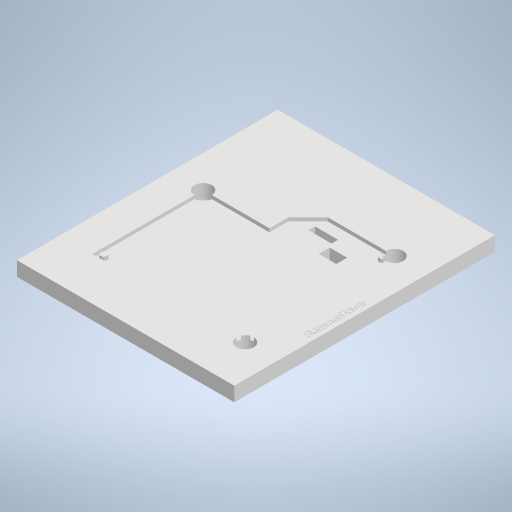
# Autodesk Inventor part: _Tooling_PCBPaste
Saved by Autodesk Inventor 2023.2 (Build 272271000, 271)
## iProperties
Created: 2023-03-08
Part Number: _Tooling_PCBPaste
Material: Generic
Document SubType Name: Modeling
Designer: atrus
Density: 1 g/cm^3
Appearance: Default
Author: atrus
Autodesk Inventor part; units mm, degrees
ref_plane "YZ Plane" through (0, 0, 0) normal (1, 0, 0) x (0, 1, 0)
ref_plane "XZ Plane" through (0, 0, 0) normal (0, 1, 0) x (-1, 0, 0)
ref_plane "XY Plane" through (0, 0, 0) normal (0, 0, 1) x (1, 0, 0)
sketch "Sketch1" plane through (0, 0, 0) normal (0, 1, 0) x (-1, 0, 0)
  line L0 (0, 0) -> (-100, 0)
  line L1 (-100, 0) -> (-100, -120)
  line L2 (-100, -120) -> (0, -120)
  line L3 (0, -120) -> (0, 0)
  dimension "d0" = 120
  dimension "d1" = 100
  constraints: 8 end point, 2 parallel, 1 horizontal, 1 perpendicular
  measures "d0" distance of L2.end L0.start
  measures "d1" distance of L0.start L0.end
extrude "Extrusion1" add sketch "Sketch1" along normal blind 5
sketch "Sketch2" plane through (0, 5, 0) normal (0, 1, 0) x (1, 0, 0)
  circle A0 centre (71.8797, 76.0683) radius 0.45 construction
  circle A1 centre (66.7997, 75.0523) radius 0.45 construction
  circle A2 centre (66.7997, 77.0843) radius 0.45 construction
  circle A3 centre (54.9887, 82.1643) radius 0.508 construction
  circle A4 centre (57.5287, 82.1643) radius 0.508 construction
  circle A5 centre (60.0687, 82.1643) radius 0.508 construction
  circle A6 centre (62.6087, 82.1643) radius 0.508 construction
  circle A7 centre (82.5477, 85.7203) radius 1.6256 construction
  circle A8 centre (82.5477, 22.7283) radius 1.6256 construction
  circle A9 centre (17.5237, 22.4743) radius 1.6256 construction
  circle A10 centre (78.7377, 80.8943) radius 0.425 construction
  circle A11 centre (66.0377, 83.4343) radius 0.425 construction
  line L0 (14.9837, 70.7343) -> (14.9837, 19.9343) construction
  line L1 (14.9837, 19.9343) -> (85.0877, 19.9343) construction
  line L2 (85.0877, 19.9343) -> (85.0877, 88.5143) construction
  line L3 (85.0877, 88.5143) -> (54.3537, 88.5143) construction
  line L4 (54.3537, 88.5143) -> (45.4637, 79.6243) construction
  line L5 (45.4637, 79.6243) -> (45.4637, 70.7343) construction
  line L6 (45.4637, 70.7343) -> (14.9837, 70.7343) construction
  line L7 (14.8837, 70.8343) -> (14.8837, 19.8343)
  line L8 (14.8837, 19.8343) -> (85.1877, 19.8343)
  line L9 (85.1877, 19.8343) -> (85.1877, 88.6143)
  line L10 (85.1877, 88.6143) -> (54.3123, 88.6143)
  line L11 (54.3123, 88.6143) -> (45.3637, 79.6658)
  line L12 (45.3637, 79.6658) -> (45.3637, 70.8343)
  line L13 (45.3637, 70.8343) -> (14.8837, 70.8343)
  circle A12 centre (82.5477, 85.7203) radius 1.5256
  circle A13 centre (17.5237, 22.4743) radius 1.5256
  circle A14 centre (82.5477, 22.7283) radius 1.5256
  line L14 (100, 120) -> (0, 120) projected
  line L15 (100, 0) -> (100, 120) projected
  line L16 (0, 120) -> (100, 120)
  line L17 (100, 120) -> (100, 0)
  line L18 (100, 0) -> (0, 0)
  line L19 (0, 0) -> (0, 120)
  point P0 (0, 0)
  dimension "d4" = 0.1
  dimension "d5" = 0.1
  dimension "d6" = 0.1
  dimension "d7" = 0.1
  constraints: 22 end point, 3 centre point, 2 parallel, 1 horizontal, 1 perpendicular, 6 other
  measures "d4" distance between parallel lines of L6 L13
  measures "d5" radial gap between concentric circles of A7 A12
  measures "d6" radial gap between concentric circles of A9 A13
  measures "d7" radial gap between concentric circles of A8 A14
extrude "Extrusion2" add sketch "Sketch2" along normal blind 1.6
sketch "Sketch3" plane through (0, 6.6, 0) normal (0, 1, 0) x (1, 0, 0)
  line L0 (45.3637, 70.8343) -> (14.8837, 70.8343) projected
  circle A0 centre (14.8837, 70.8343) radius 4
  line L1 (85.1877, 88.6143) -> (54.3123, 88.6143) projected
  circle A1 centre (85.1877, 88.6143) radius 4
  line L2 (85.1877, 19.8343) -> (14.8837, 19.8343) projected
  circle A2 centre (85.1877, 19.8343) radius 4
  circle A3 centre (54.9887, 82.1643) radius 0.508 construction
  circle A4 centre (62.6087, 82.1643) radius 0.508 construction
  circle A5 centre (66.7997, 77.0843) radius 0.45 construction
  circle A6 centre (71.8797, 76.0683) radius 0.45 construction
  circle A7 centre (66.7997, 75.0523) radius 0.45 construction
  line L3 (53.4887, 83.6643) -> (64.1087, 83.6643)
  line L4 (64.1087, 83.6643) -> (64.1087, 80.6643)
  line L5 (64.1087, 80.6643) -> (53.4887, 80.6643)
  line L6 (53.4887, 80.6643) -> (53.4887, 83.6643)
  line L7 (65.2997, 78.5843) -> (73.3797, 78.5843)
  line L8 (73.3797, 78.5843) -> (73.3797, 73.5523)
  line L9 (73.3797, 73.5523) -> (65.2997, 73.5523)
  line L10 (65.2997, 73.5523) -> (65.2997, 78.5843)
  point P0 (0, 0)
  point P1 (53.4887, 82.1643)
  point P2 (64.1087, 82.1643)
  point P3 (73.3797, 76.0683)
  dimension "d10" = 8
  dimension "d11" = 1.5
  dimension "d12" = 1.5
  dimension "d13" = 1.5
  dimension "d14" = 1.5
  dimension "d15" = 1.5
  dimension "d16" = 1.5
  dimension "d17" = 1.5
  dimension "d18" = 1.5
  constraints: 16 end point, 4 parallel, 3 centre point, 3 midpoint, 2 equal radius, 2 horizontal, 2 perpendicular
  measures "d10" diameter of A0
  measures "d11" distance of point (53.489, 82.164) A3.centre
  measures "d12" distance of point (64.109, 82.164) A4.centre
  measures "d13" distance from line of L5 A4.centre
  measures "d14" distance from line of L3 A3.centre
  measures "d15" distance from line of L7 A5.centre
  measures "d16" distance from line of L9 A7.centre
  measures "d17" distance from line of L10 A7.centre
  measures "d18" distance of point (73.38, 76.068) A6.centre
extrude "Extrusion3" cut sketch "Sketch3" against normal through all
sketch "Sketch4" plane through (0, 6.6, 0) normal (0, 1, 0) x (1, 0, 0)
  line L0 (94.8886, 36.1606) -> (94.8886, 63.4147) construction
  line L1 (94.8886, 63.4147) -> (98.1268, 63.4147) construction
  line L2 (98.1268, 63.4147) -> (98.1268, 36.1606) construction
  line L3 (98.1268, 36.1606) -> (94.8886, 36.1606) construction
  spline S0 degree 2 poles (98.1268, 37.319) (98.1268, 36.988) (97.9885, 36.5237) (97.8897, 36.3186) knots 0 0 0 1 2 2 2
  line L4 (97.8897, 36.3186) -> (97.3809, 36.3186)
  line L5 (97.3809, 36.3186) -> (97.3809, 36.3483)
  spline S1 degree 2 poles (97.3809, 36.3483) (97.5686, 36.5484) (97.7761, 37.0547) (97.7761, 37.2894) knots 0 0 0 1 2 2 2
  spline S2 degree 2 poles (97.7761, 37.2894) (97.7761, 37.6253) (97.4969, 37.9686) (97.2672, 37.9686) knots 0 0 0 1 2 2 2
  spline S3 degree 2 poles (97.2672, 37.9686) (97.0845, 37.9686) (96.8572, 37.7883) (96.8004, 37.5932) knots 0 0 0 1 2 2 2
  spline S4 degree 2 poles (96.8004, 37.5932) (96.7609, 37.4524) (96.7065, 37.2177) (96.6621, 37.0424) knots 0 0 0 1 2 2 2
  spline S5 degree 2 poles (96.6621, 37.0424) (96.6201, 36.8843) (96.4941, 36.6348) (96.3928, 36.5385) knots 0 0 0 1 2 2 2
  spline S6 degree 2 poles (96.3928, 36.5385) (96.2916, 36.4446) (96.0199, 36.3409) (95.842, 36.3409) knots 0 0 0 1 2 2 2
  spline S7 degree 2 poles (95.842, 36.3409) (95.4715, 36.3409) (94.9701, 36.9189) (94.9701, 37.3659) knots 0 0 0 1 2 2 2
  spline S8 degree 2 poles (94.9701, 37.3659) (94.9701, 37.6228) (95.0714, 38.0773) (95.1677, 38.2724) knots 0 0 0 1 2 2 2
  line L6 (95.1677, 38.2724) -> (95.6518, 38.2724)
  line L7 (95.6518, 38.2724) -> (95.6518, 38.2428)
  spline S9 degree 2 poles (95.6518, 38.2428) (95.5185, 38.0971) (95.3209, 37.6426) (95.3209, 37.3931) knots 0 0 0 1 2 2 2
  spline S10 degree 2 poles (95.3209, 37.3931) (95.3209, 37.1115) (95.5852, 36.7632) (95.8, 36.7632) knots 0 0 0 1 2 2 2
  spline S11 degree 2 poles (95.8, 36.7632) (95.9927, 36.7632) (96.2224, 36.9683) (96.2743, 37.1609) knots 0 0 0 1 2 2 2
  spline S12 degree 2 poles (96.2743, 37.1609) (96.3089, 37.2894) (96.3978, 37.6623) (96.4348, 37.7858) knots 0 0 0 1 2 2 2
  spline S13 degree 2 poles (96.4348, 37.7858) (96.5312, 38.0995) (96.919, 38.391) (97.203, 38.391) knots 0 0 0 1 2 2 2
  spline S14 degree 2 poles (97.203, 38.391) (97.3833, 38.391) (97.7291, 38.2453) (97.8502, 38.1143) knots 0 0 0 1 2 2 2
  spline S15 degree 2 poles (97.8502, 38.1143) (97.9835, 37.9686) (98.1268, 37.5981) (98.1268, 37.319) knots 0 0 0 1 2 2 2
  line L8 (98.0725, 40.6683) -> (98.0725, 40.162)
  line L9 (98.0725, 40.162) -> (96.9684, 39.3123)
  line L10 (96.9684, 39.3123) -> (97.1166, 39.1592)
  line L11 (97.1166, 39.1592) -> (98.0725, 39.1592)
  line L12 (98.0725, 39.1592) -> (98.0725, 38.7738)
  line L13 (98.0725, 38.7738) -> (94.8886, 38.7738)
  line L14 (94.8886, 38.7738) -> (94.8886, 39.1592)
  line L15 (94.8886, 39.1592) -> (96.751, 39.1592)
  line L16 (96.751, 39.1592) -> (95.7852, 40.0632)
  line L17 (95.7852, 40.0632) -> (95.7852, 40.5424)
  line L18 (95.7852, 40.5424) -> (96.7411, 39.6038)
  line L19 (96.7411, 39.6038) -> (98.0725, 40.6683)
  line L20 (98.0725, 41.2537) -> (98.0725, 40.8684)
  line L21 (98.0725, 40.8684) -> (95.7852, 40.8684)
  line L22 (95.7852, 40.8684) -> (95.7852, 41.2537)
  line L23 (95.7852, 41.2537) -> (98.0725, 41.2537)
  line L24 (95.4048, 41.2809) -> (95.4048, 40.8437)
  line L25 (95.4048, 40.8437) -> (95.0047, 40.8437)
  line L26 (95.0047, 40.8437) -> (95.0047, 41.2809)
  line L27 (95.0047, 41.2809) -> (95.4048, 41.2809)
  line L28 (98.0725, 44.4129) -> (96.7485, 44.4129)
  spline S16 degree 2 poles (96.7485, 44.4129) (96.5904, 44.4129) (96.3212, 44.3882) (96.2471, 44.3487) knots 0 0 0 1 2 2 2
  spline S17 degree 2 poles (96.2471, 44.3487) (96.1656, 44.3091) (96.0866, 44.1585) (96.0866, 44.0276) knots 0 0 0 1 2 2 2
  spline S18 degree 2 poles (96.0866, 44.0276) (96.0866, 43.909) (96.2323, 43.6373) (96.3706, 43.494) knots 0 0 0 1 2 2 2
  spline S19 degree 2 poles (96.3706, 43.494) (96.4052, 43.4965) (96.5015, 43.5014) (96.5657, 43.5014) knots 0 0 0 1 2 2 2
  line L29 (96.5657, 43.5014) -> (98.0725, 43.5014)
  line L30 (98.0725, 43.5014) -> (98.0725, 43.1161)
  line L31 (98.0725, 43.1161) -> (96.7485, 43.1161)
  spline S20 degree 2 poles (96.7485, 43.1161) (96.5904, 43.1161) (96.3212, 43.0914) (96.2471, 43.0519) knots 0 0 0 1 2 2 2
  spline S21 degree 2 poles (96.2471, 43.0519) (96.1656, 43.0124) (96.0866, 42.8617) (96.0866, 42.7308) knots 0 0 0 1 2 2 2
  spline S22 degree 2 poles (96.0866, 42.7308) (96.0866, 42.6073) (96.2422, 42.3331) (96.3632, 42.2047) knots 0 0 0 1 2 2 2
  line L32 (96.3632, 42.2047) -> (98.0725, 42.2047)
  line L33 (98.0725, 42.2047) -> (98.0725, 41.8194)
  line L34 (98.0725, 41.8194) -> (95.7852, 41.8194)
  line L35 (95.7852, 41.8194) -> (95.7852, 42.2047)
  line L36 (95.7852, 42.2047) -> (96.0372, 42.2047)
  spline S23 degree 2 poles (96.0372, 42.2047) (95.8865, 42.3554) (95.721, 42.6518) (95.721, 42.8296) knots 0 0 0 1 2 2 2
  spline S24 degree 2 poles (95.721, 42.8296) (95.721, 43.0321) (95.9063, 43.3458) (96.1162, 43.4273) knots 0 0 0 1 2 2 2
  spline S25 degree 2 poles (96.1162, 43.4273) (95.9211, 43.6027) (95.721, 43.9337) (95.721, 44.1264) knots 0 0 0 1 2 2 2
  spline S26 degree 2 poles (95.721, 44.1264) (95.721, 44.2746) (95.8124, 44.5166) (95.9161, 44.6055) knots 0 0 0 1 2 2 2
  spline S27 degree 2 poles (95.9161, 44.6055) (96.0199, 44.6969) (96.3311, 44.7982) (96.5657, 44.7982) knots 0 0 0 1 2 2 2
  line L37 (96.5657, 44.7982) -> (98.0725, 44.7982)
  line L38 (98.0725, 44.7982) -> (98.0725, 44.4129)
  line L39 (98.0725, 47.9327) -> (96.7485, 47.9327)
  spline S28 degree 2 poles (96.7485, 47.9327) (96.5904, 47.9327) (96.3212, 47.908) (96.2471, 47.8684) knots 0 0 0 1 2 2 2
  spline S29 degree 2 poles (96.2471, 47.8684) (96.1656, 47.8289) (96.0866, 47.6782) (96.0866, 47.5473) knots 0 0 0 1 2 2 2
  spline S30 degree 2 poles (96.0866, 47.5473) (96.0866, 47.4288) (96.2323, 47.1571) (96.3706, 47.0138) knots 0 0 0 1 2 2 2
  spline S31 degree 2 poles (96.3706, 47.0138) (96.4052, 47.0163) (96.5015, 47.0212) (96.5657, 47.0212) knots 0 0 0 1 2 2 2
  line L40 (96.5657, 47.0212) -> (98.0725, 47.0212)
  line L41 (98.0725, 47.0212) -> (98.0725, 46.6359)
  line L42 (98.0725, 46.6359) -> (96.7485, 46.6359)
  spline S32 degree 2 poles (96.7485, 46.6359) (96.5904, 46.6359) (96.3212, 46.6112) (96.2471, 46.5717) knots 0 0 0 1 2 2 2
  spline S33 degree 2 poles (96.2471, 46.5717) (96.1656, 46.5322) (96.0866, 46.3815) (96.0866, 46.2506) knots 0 0 0 1 2 2 2
  spline S34 degree 2 poles (96.0866, 46.2506) (96.0866, 46.1271) (96.2422, 45.8529) (96.3632, 45.7245) knots 0 0 0 1 2 2 2
  line L43 (96.3632, 45.7245) -> (98.0725, 45.7245)
  line L44 (98.0725, 45.7245) -> (98.0725, 45.3391)
  line L45 (98.0725, 45.3391) -> (95.7852, 45.3391)
  line L46 (95.7852, 45.3391) -> (95.7852, 45.7245)
  line L47 (95.7852, 45.7245) -> (96.0372, 45.7245)
  spline S35 degree 2 poles (96.0372, 45.7245) (95.8865, 45.8751) (95.721, 46.1715) (95.721, 46.3494) knots 0 0 0 1 2 2 2
  spline S36 degree 2 poles (95.721, 46.3494) (95.721, 46.5519) (95.9063, 46.8656) (96.1162, 46.9471) knots 0 0 0 1 2 2 2
  spline S37 degree 2 poles (96.1162, 46.9471) (95.9211, 47.1225) (95.721, 47.4535) (95.721, 47.6461) knots 0 0 0 1 2 2 2
  spline S38 degree 2 poles (95.721, 47.6461) (95.721, 47.7943) (95.8124, 48.0364) (95.9161, 48.1253) knots 0 0 0 1 2 2 2
  spline S39 degree 2 poles (95.9161, 48.1253) (96.0199, 48.2167) (96.3311, 48.318) (96.5657, 48.318) knots 0 0 0 1 2 2 2
  line L48 (96.5657, 48.318) -> (98.0725, 48.318)
  line L49 (98.0725, 48.318) -> (98.0725, 47.9327)
  spline S40 degree 2 poles (98.1243, 49.8519) (98.1243, 49.3035) (97.5093, 48.7008) (96.9412, 48.7008) knots 0 0 0 1 2 2 2
  spline S41 degree 2 poles (96.9412, 48.7008) (96.383, 48.7008) (95.721, 49.2862) (95.721, 49.758) knots 0 0 0 1 2 2 2
  spline S42 degree 2 poles (95.721, 49.758) (95.721, 49.9704) (95.8445, 50.2989) (95.9754, 50.42) knots 0 0 0 1 2 2 2
  spline S43 degree 2 poles (95.9754, 50.42) (96.1063, 50.5435) (96.4842, 50.6744) (96.7584, 50.6744) knots 0 0 0 1 2 2 2
  line L50 (96.7584, 50.6744) -> (96.9684, 50.6744)
  line L51 (96.9684, 50.6744) -> (96.9684, 49.0911)
  spline S44 degree 2 poles (96.9684, 49.0911) (97.366, 49.0911) (97.7884, 49.4912) (97.7884, 49.8469) knots 0 0 0 1 2 2 2
  spline S45 degree 2 poles (97.7884, 49.8469) (97.7884, 49.9729) (97.7316, 50.2174) (97.6871, 50.3162) knots 0 0 0 1 2 2 2
  spline S46 degree 2 poles (97.6871, 50.3162) (97.6377, 50.42) (97.5513, 50.5632) (97.5118, 50.6102) knots 0 0 0 1 2 2 2
  line L52 (97.5118, 50.6102) -> (97.5118, 50.6324)
  line L53 (97.5118, 50.6324) -> (97.9317, 50.6324)
  spline S47 degree 2 poles (97.9317, 50.6324) (97.9588, 50.5657) (98.0379, 50.3632) (98.0601, 50.2841) knots 0 0 0 1 2 2 2
  spline S48 degree 2 poles (98.0601, 50.2841) (98.0922, 50.173) (98.1243, 49.9902) (98.1243, 49.8519) knots 0 0 0 1 2 2 2
  spline S49 degree 2 poles (96.6744, 50.2989) (96.5188, 50.294) (96.2916, 50.2298) (96.215, 50.168) knots 0 0 0 1 2 2 2
  spline S50 degree 2 poles (96.215, 50.168) (96.1286, 50.1013) (96.0372, 49.8914) (96.0372, 49.7358) knots 0 0 0 1 2 2 2
  spline S51 degree 2 poles (96.0372, 49.7358) (96.0372, 49.5826) (96.1286, 49.3677) (96.2175, 49.2788) knots 0 0 0 1 2 2 2
  spline S52 degree 2 poles (96.2175, 49.2788) (96.3089, 49.1924) (96.5287, 49.1034) (96.6744, 49.0911) knots 0 0 0 1 2 2 2
  line L54 (96.6744, 49.0911) -> (96.6744, 50.2989)
  line L55 (96.1977, 52.2774) -> (96.1977, 52.2577)
  spline S53 degree 2 poles (96.1977, 52.2577) (96.1854, 52.2132) (96.1804, 52.1169) (96.1804, 52.0502) knots 0 0 0 1 2 2 2
  spline S54 degree 2 poles (96.1804, 52.0502) (96.1804, 51.8946) (96.3163, 51.5883) (96.4497, 51.45) knots 0 0 0 1 2 2 2
  line L56 (96.4497, 51.45) -> (98.0725, 51.45)
  line L57 (98.0725, 51.45) -> (98.0725, 51.0646)
  line L58 (98.0725, 51.0646) -> (95.7852, 51.0646)
  line L59 (95.7852, 51.0646) -> (95.7852, 51.45)
  line L60 (95.7852, 51.45) -> (96.1261, 51.45)
  spline S55 degree 2 poles (96.1261, 51.45) (95.9384, 51.6599) (95.7852, 51.9736) (95.7852, 52.1218) knots 0 0 0 1 2 2 2
  spline S56 degree 2 poles (95.7852, 52.1218) (95.7852, 52.1811) (95.7902, 52.2404) (95.7976, 52.2774) knots 0 0 0 1 2 2 2
  line L61 (95.7976, 52.2774) -> (96.1977, 52.2774)
  spline S57 degree 2 poles (96.5509, 55.0093) (96.9684, 55.0093) (97.6402, 54.6709) (97.8279, 54.3868) knots 0 0 0 1 2 2 2
  spline S58 degree 2 poles (97.8279, 54.3868) (97.9737, 54.1546) (98.0725, 53.6779) (98.0725, 53.3074) knots 0 0 0 1 2 2 2
  line L62 (98.0725, 53.3074) -> (98.0725, 52.6059)
  line L63 (98.0725, 52.6059) -> (95.0245, 52.6059)
  line L64 (95.0245, 52.6059) -> (95.0245, 53.3)
  spline S59 degree 2 poles (95.0245, 53.3) (95.0245, 53.7298) (95.1529, 54.2188) (95.2665, 54.3918) knots 0 0 0 1 2 2 2
  spline S60 degree 2 poles (95.2665, 54.3918) (95.4617, 54.6857) (96.1063, 55.0093) (96.5509, 55.0093) knots 0 0 0 1 2 2 2
  spline S61 degree 2 poles (96.546, 54.5869) (96.1952, 54.5869) (95.6988, 54.3547) (95.558, 54.125) knots 0 0 0 1 2 2 2
  spline S62 degree 2 poles (95.558, 54.125) (95.4617, 53.962) (95.3752, 53.5939) (95.3752, 53.3198) knots 0 0 0 1 2 2 2
  line L65 (95.3752, 53.3198) -> (95.3752, 53.011)
  line L66 (95.3752, 53.011) -> (97.7217, 53.011)
  line L67 (97.7217, 53.011) -> (97.7217, 53.3198)
  spline S63 degree 2 poles (97.7217, 53.3198) (97.7217, 53.589) (97.6353, 53.9965) (97.5192, 54.162) knots 0 0 0 1 2 2 2
  spline S64 degree 2 poles (97.5192, 54.162) (97.3759, 54.3745) (96.9017, 54.5869) (96.546, 54.5869) knots 0 0 0 1 2 2 2
  line L68 (96.1977, 56.6321) -> (96.1977, 56.6123)
  spline S65 degree 2 poles (96.1977, 56.6123) (96.1854, 56.5678) (96.1804, 56.4715) (96.1804, 56.4048) knots 0 0 0 1 2 2 2
  spline S66 degree 2 poles (96.1804, 56.4048) (96.1804, 56.2492) (96.3163, 55.9429) (96.4497, 55.8046) knots 0 0 0 1 2 2 2
  line L69 (96.4497, 55.8046) -> (98.0725, 55.8046)
  line L70 (98.0725, 55.8046) -> (98.0725, 55.4193)
  line L71 (98.0725, 55.4193) -> (95.7852, 55.4193)
  line L72 (95.7852, 55.4193) -> (95.7852, 55.8046)
  line L73 (95.7852, 55.8046) -> (96.1261, 55.8046)
  spline S67 degree 2 poles (96.1261, 55.8046) (95.9384, 56.0146) (95.7852, 56.3282) (95.7852, 56.4764) knots 0 0 0 1 2 2 2
  spline S68 degree 2 poles (95.7852, 56.4764) (95.7852, 56.5357) (95.7902, 56.595) (95.7976, 56.6321) knots 0 0 0 1 2 2 2
  line L74 (95.7976, 56.6321) -> (96.1977, 56.6321)
  line L75 (98.0725, 57.3237) -> (98.0725, 56.9383)
  line L76 (98.0725, 56.9383) -> (95.7852, 56.9383)
  line L77 (95.7852, 56.9383) -> (95.7852, 57.3237)
  line L78 (95.7852, 57.3237) -> (98.0725, 57.3237)
  line L79 (95.4048, 57.3508) -> (95.4048, 56.9136)
  line L80 (95.4048, 56.9136) -> (95.0047, 56.9136)
  line L81 (95.0047, 56.9136) -> (95.0047, 57.3508)
  line L82 (95.0047, 57.3508) -> (95.4048, 57.3508)
  line L83 (95.7852, 59.685) -> (98.0725, 58.823)
  line L84 (98.0725, 58.823) -> (98.0725, 58.4772)
  line L85 (98.0725, 58.4772) -> (95.7852, 57.6225)
  line L86 (95.7852, 57.6225) -> (95.7852, 58.04)
  line L87 (95.7852, 58.04) -> (97.5463, 58.6649)
  line L88 (97.5463, 58.6649) -> (95.7852, 59.2849)
  line L89 (95.7852, 59.2849) -> (95.7852, 59.685)
  spline S69 degree 2 poles (98.1243, 60.9694) (98.1243, 60.4211) (97.5093, 59.8184) (96.9412, 59.8184) knots 0 0 0 1 2 2 2
  spline S70 degree 2 poles (96.9412, 59.8184) (96.383, 59.8184) (95.721, 60.4038) (95.721, 60.8755) knots 0 0 0 1 2 2 2
  spline S71 degree 2 poles (95.721, 60.8755) (95.721, 61.088) (95.8445, 61.4165) (95.9754, 61.5375) knots 0 0 0 1 2 2 2
  spline S72 degree 2 poles (95.9754, 61.5375) (96.1063, 61.661) (96.4842, 61.7919) (96.7584, 61.7919) knots 0 0 0 1 2 2 2
  line L90 (96.7584, 61.7919) -> (96.9684, 61.7919)
  line L91 (96.9684, 61.7919) -> (96.9684, 60.2086)
  spline S73 degree 2 poles (96.9684, 60.2086) (97.366, 60.2086) (97.7884, 60.6088) (97.7884, 60.9645) knots 0 0 0 1 2 2 2
  spline S74 degree 2 poles (97.7884, 60.9645) (97.7884, 61.0904) (97.7316, 61.335) (97.6871, 61.4338) knots 0 0 0 1 2 2 2
  spline S75 degree 2 poles (97.6871, 61.4338) (97.6377, 61.5375) (97.5513, 61.6808) (97.5118, 61.7277) knots 0 0 0 1 2 2 2
  line L92 (97.5118, 61.7277) -> (97.5118, 61.7499)
  line L93 (97.5118, 61.7499) -> (97.9317, 61.7499)
  spline S76 degree 2 poles (97.9317, 61.7499) (97.9588, 61.6832) (98.0379, 61.4807) (98.0601, 61.4017) knots 0 0 0 1 2 2 2
  spline S77 degree 2 poles (98.0601, 61.4017) (98.0922, 61.2905) (98.1243, 61.1077) (98.1243, 60.9694) knots 0 0 0 1 2 2 2
  spline S78 degree 2 poles (96.6744, 61.4165) (96.5188, 61.4115) (96.2916, 61.3473) (96.215, 61.2856) knots 0 0 0 1 2 2 2
  spline S79 degree 2 poles (96.215, 61.2856) (96.1286, 61.2189) (96.0372, 61.0089) (96.0372, 60.8533) knots 0 0 0 1 2 2 2
  spline S80 degree 2 poles (96.0372, 60.8533) (96.0372, 60.7002) (96.1286, 60.4853) (96.2175, 60.3964) knots 0 0 0 1 2 2 2
  spline S81 degree 2 poles (96.2175, 60.3964) (96.3089, 60.3099) (96.5287, 60.221) (96.6744, 60.2086) knots 0 0 0 1 2 2 2
  line L94 (96.6744, 60.2086) -> (96.6744, 61.4165)
  line L95 (96.1977, 63.395) -> (96.1977, 63.3752)
  spline S82 degree 2 poles (96.1977, 63.3752) (96.1854, 63.3307) (96.1804, 63.2344) (96.1804, 63.1677) knots 0 0 0 1 2 2 2
  spline S83 degree 2 poles (96.1804, 63.1677) (96.1804, 63.0121) (96.3163, 62.7058) (96.4497, 62.5675) knots 0 0 0 1 2 2 2
  line L96 (96.4497, 62.5675) -> (98.0725, 62.5675)
  line L97 (98.0725, 62.5675) -> (98.0725, 62.1822)
  line L98 (98.0725, 62.1822) -> (95.7852, 62.1822)
  line L99 (95.7852, 62.1822) -> (95.7852, 62.5675)
  line L100 (95.7852, 62.5675) -> (96.1261, 62.5675)
  spline S84 degree 2 poles (96.1261, 62.5675) (95.9384, 62.7775) (95.7852, 63.0911) (95.7852, 63.2393) knots 0 0 0 1 2 2 2
  spline S85 degree 2 poles (95.7852, 63.2393) (95.7852, 63.2986) (95.7902, 63.3579) (95.7976, 63.395) knots 0 0 0 1 2 2 2
  line L101 (95.7976, 63.395) -> (96.1977, 63.395)
  point P0 (0, 0)
  constraints: 2 other
emboss "Emboss1" sketch "Sketch4" operation cut depth 0.2 direction (0, -1, 0)
body "Solid1"
